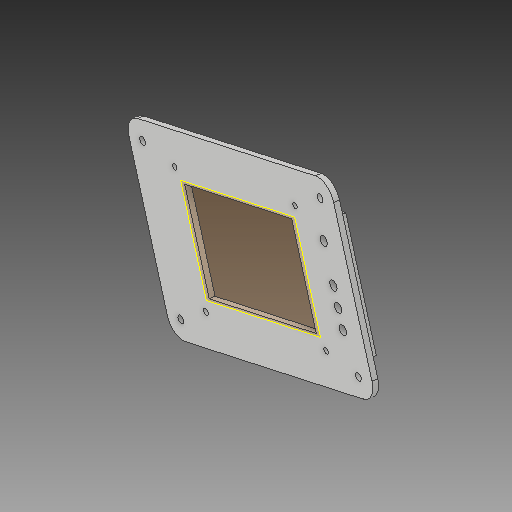
# Autodesk Inventor part: Tampa Painel
Saved by Autodesk Inventor 2019 (Build 230136000, 136)
## iProperties
Created: 2020-05-29
Part Number: Tampa Painel
Material: Generic
Document SubType Name: Modeling
Designer: luiza
Density: 1 g/cm^3
Appearance: Default
Author: luiza
Autodesk Inventor part; units mm, degrees
ref_plane "YZ Plane" through (0, 0, 0) normal (1, 0, 0) x (0, 1, 0)
ref_plane "XZ Plane" through (0, 0, 0) normal (0, 1, 0) x (-1, 0, 0)
ref_plane "XY Plane" through (0, 0, 0) normal (0, 0, 1) x (1, 0, 0)
ref_plane "Work Plane2" through (-1670.9187, -273.4985, -5718.1339) normal (-0.1475237, -0.0099436, 0.9890085) x (0.9373069, 0.3178125, 0.143007)
sketch "Sketch2" plane through (-1670.9187, -273.4985, -5718.1339) normal (-0.1475237, -0.0099436, 0.9890085) x (0.9373069, 0.3178125, 0.143007)
  line L0 (0, 51) -> (78, 51) construction
  line L1 (78, 51) -> (78, 0) construction
  line L2 (78, 0) -> (0, 0) construction
  line L3 (0, 0) -> (0, 51) construction
  line L4 (78.2, 51.2) -> (-0.2, 51.2)
  line L5 (-0.2, 51.2) -> (-0.2, -0.2)
  line L6 (-0.2, -0.2) -> (78.2, -0.2)
  line L7 (78.2, -0.2) -> (78.2, 51.2)
  line L8 (-26, 75.5) -> (104, 75.5)
  line L9 (114, 65.5) -> (114, -14.5)
  line L10 (-26, -24.5) -> (104, -24.5)
  line L11 (-36, 65.5) -> (-36, -14.5)
  line L12 (-7.5, 75.5) -> (-7.5, -24.5) construction
  circle A0 centre (1109.8895, -39.0871) radius 1.5 projected
  circle A1 centre (1103.525, -103.7747) radius 1.5 projected
  circle A2 centre (1191.1021, -112.3913) radius 1.5 projected
  circle A3 centre (1197.4666, -47.7037) radius 1.5 projected
  arc A4 (-26, 75.5) -> (-36, 65.5) centre (-26, 65.5) ccw
  arc A5 (114, 65.5) -> (104, 75.5) centre (104, 65.5) ccw
  arc A6 (104, -24.5) -> (114, -14.5) centre (104, -14.5) ccw
  arc A7 (-36, -14.5) -> (-26, -24.5) centre (-26, -14.5) ccw
  circle A8 centre (99.75, 5.5) radius 2.5
  circle A9 centre (99.75, 15.5) radius 2.5
  circle A10 centre (99.75, 25.5) radius 2.5
  circle A11 centre (99.6463, 45.4997) radius 2.5
  point P0 (2470.8183, -483.0734)
  point P1 (114, 75.5)
  point P2 (114, -24.5)
  point P3 (114, 25.5)
  point P4 (78, 25.5)
  point P5 (-36, 75.5)
  point P6 (-36, -24.5)
  point P7 (39, 75.5)
  point P8 (39, 51)
  dimension "d1" = 0.2
  dimension "d3" = 100
  dimension "d4" = 150
  dimension "d12" = 10
  dimension "d17" = 5
  dimension "d18" = 5
  dimension "d19" = 5
  dimension "d21" = 5
  dimension "d22" = 5
  dimension "d23" = 14.25
  dimension "d24" = 40
  dimension "d27" = 5
  dimension "d29" = 15
  constraints: 26 end point, 10 point on line, 8 centre point, 8 point on circle, 8 tangent, 4 midpoint, 4 parallel, 3 equal radius, 3 horizontal, 3 perpendicular, 2 vertical, 1 horizontal alignment, 1 vertical alignment, 5 other
  measures "d1" distance between parallel lines of L0 L4
  measures "d3" distance between parallel lines of L8 L10
  measures "d4" distance between parallel lines of L11 L9
  measures "d12" radius of A4
  measures "d17" diameter of A10
  measures "d18" diameter of A9
  measures "d19" diameter of A8
  measures "d23" distance from line of L9 A9.centre
  measures "d24" distance from line of L10 A9.centre
  measures "d27" diameter of A11
extrude "Extrusion2" add sketch "Sketch2" against normal blind 3 contours L8 A5 L9 A6 L10 A7 L11 A4
sketch "Sketch3" plane through (-1670.9187, -273.4985, -5718.1339) normal (-0.1475237, -0.0099436, 0.9890085) x (0.9373069, 0.3178125, 0.143007)
  line L0 (-26, -7.5) -> (-33, -7.5) projected
  line L1 (-33, -7.5) -> (-33, 58.5) projected
  line L2 (-33, 58.5) -> (-26, 58.5) projected
  line L3 (-19, 65.5) -> (-19, 72.5) projected
  line L4 (-19, 72.5) -> (97, 72.5) projected
  line L5 (97, 72.5) -> (97, 65.5) projected
  line L6 (104, 58.5) -> (111, 58.5) projected
  line L7 (111, 58.5) -> (111, -7.5) projected
  line L8 (111, -7.5) -> (104, -7.5) projected
  line L9 (97, -14.5) -> (97, -21.5) projected
  line L10 (97, -21.5) -> (-19, -21.5) projected
  line L11 (-19, -21.5) -> (-19, -14.5) projected
  line L12 (-36, -14.5) -> (-36, 65.5) projected
  line L13 (104, -24.5) -> (-26, -24.5) projected
  line L14 (114, 65.5) -> (114, -14.5) projected
  line L15 (-26, 75.5) -> (104, 75.5) projected
  circle A0 centre (-26, 65.5) radius 2 projected
  circle A1 centre (104, -14.5) radius 2 projected
  circle A2 centre (-26, -14.5) radius 2 projected
  circle A3 centre (104, 65.5) radius 2 projected
  arc A4 (-26, 58.5) -> (-19, 65.5) centre (-26, 65.5) ccw projected
  arc A5 (97, 65.5) -> (104, 58.5) centre (104, 65.5) ccw projected
  arc A6 (104, -7.5) -> (97, -14.5) centre (104, -14.5) ccw projected
  arc A7 (-19, -14.5) -> (-26, -7.5) centre (-26, -14.5) ccw projected
  arc A8 (-36, -14.5) -> (-26, -24.5) centre (-26, -14.5) ccw projected
  arc A9 (104, -24.5) -> (114, -14.5) centre (104, -14.5) ccw projected
  arc A10 (114, 65.5) -> (104, 75.5) centre (104, 65.5) ccw projected
  arc A11 (-26, 75.5) -> (-36, 65.5) centre (-26, 65.5) ccw projected
  point P0 (2470.8183, -483.0734)
extrude "Extrusion3" cut sketch "Sketch3" against normal through all contours A0 | A1 | A2 | A3
sketch "Sketch4" plane through (-1670.4761, -273.4687, -5721.1009) normal (0.1475237, 0.0099436, -0.9890085) x (-0.9373069, -0.3178125, -0.143007)
  line L0 (26, -7.5) -> (33, -7.5) projected
  line L1 (33, -7.5) -> (33, 58.5) projected
  line L2 (33, 58.5) -> (26, 58.5) projected
  line L3 (19, 65.5) -> (19, 72.5) projected
  line L4 (19, 72.5) -> (-97, 72.5) projected
  line L5 (-97, 72.5) -> (-97, 65.5) projected
  line L6 (-104, 58.5) -> (-111, 58.5) projected
  line L7 (-111, 58.5) -> (-111, -7.5) projected
  line L8 (-111, -7.5) -> (-104, -7.5) projected
  line L9 (-97, -14.5) -> (-97, -21.5) projected
  line L10 (-97, -21.5) -> (19, -21.5) projected
  line L11 (19, -21.5) -> (19, -14.5) projected
  line L12 (36, -14.5) -> (36, 65.5) projected
  line L13 (-104, -24.5) -> (26, -24.5) projected
  line L14 (-114, 65.5) -> (-114, -14.5) projected
  line L15 (26, 75.5) -> (-104, 75.5) projected
  circle A0 centre (26, 65.5) radius 2 projected
  circle A1 centre (-104, -14.5) radius 2 projected
  circle A2 centre (26, -14.5) radius 2 projected
  circle A3 centre (-104, 65.5) radius 2 projected
  arc A4 (19, 65.5) -> (26, 58.5) centre (26, 65.5) ccw projected
  arc A5 (-104, 58.5) -> (-97, 65.5) centre (-104, 65.5) ccw projected
  arc A6 (-97, -14.5) -> (-104, -7.5) centre (-104, -14.5) ccw projected
  arc A7 (26, -7.5) -> (19, -14.5) centre (26, -14.5) ccw projected
  arc A8 (26, -24.5) -> (36, -14.5) centre (26, -14.5) ccw projected
  arc A9 (-114, -14.5) -> (-104, -24.5) centre (-104, -14.5) ccw projected
  arc A10 (-104, 75.5) -> (-114, 65.5) centre (-104, 65.5) ccw projected
  arc A11 (36, 65.5) -> (26, 75.5) centre (26, 65.5) ccw projected
  line L16 (-96, 65.5) -> (-96, 71.5)
  line L17 (-96, 71.5) -> (18, 71.5)
  line L18 (18, 71.5) -> (18, 65.5)
  arc A12 (18, 65.5) -> (26, 57.5) centre (26, 65.5) ccw
  line L19 (26, 57.5) -> (32, 57.5)
  line L20 (32, 57.5) -> (32, -6.5)
  line L21 (32, -6.5) -> (26, -6.5)
  arc A13 (26, -6.5) -> (18, -14.5) centre (26, -14.5) ccw
  line L22 (18, -14.5) -> (18, -20.5)
  line L23 (18, -20.5) -> (-96, -20.5)
  line L24 (-96, -20.5) -> (-96, -14.5)
  arc A14 (-96, -14.5) -> (-104, -6.5) centre (-104, -14.5) ccw
  line L25 (-104, -6.5) -> (-110, -6.5)
  line L26 (-110, -6.5) -> (-110, 57.5)
  line L27 (-110, 57.5) -> (-104, 57.5)
  arc A15 (-104, 57.5) -> (-96, 65.5) centre (-104, 65.5) ccw
  line L28 (-93, 65.5) -> (-93, 68.5)
  line L29 (-93, 68.5) -> (15, 68.5)
  line L30 (15, 68.5) -> (15, 65.5)
  arc A16 (15, 65.5) -> (26, 54.5) centre (26, 65.5) ccw
  line L31 (26, 54.5) -> (29, 54.5)
  line L32 (29, 54.5) -> (29, -3.5)
  line L33 (29, -3.5) -> (26, -3.5)
  arc A17 (26, -3.5) -> (15, -14.5) centre (26, -14.5) ccw
  line L34 (15, -14.5) -> (15, -17.5)
  line L35 (15, -17.5) -> (-93, -17.5)
  line L36 (-93, -17.5) -> (-93, -14.5)
  arc A18 (-93, -14.5) -> (-104, -3.5) centre (-104, -14.5) ccw
  line L37 (-104, -3.5) -> (-107, -3.5)
  line L38 (-107, -3.5) -> (-107, 54.5)
  line L39 (-107, 54.5) -> (-104, 54.5)
  arc A19 (-104, 54.5) -> (-93, 65.5) centre (-104, 65.5) ccw
  point P0 (-2470.8183, -483.0734)
  point P1 (26, 65.5)
  point P2 (-104, 65.5)
  point P3 (-104, -14.5)
  point P4 (26, -14.5)
  dimension "d38" = 1
  dimension "d39" = 3
  constraints: 48 end point, 16 point on circle, 8 centre point, 30 other
  measures "d38" radial gap between concentric circles of A5 A15
  measures "d39" radial gap between concentric circles of A15 A19
extrude "Extrusion4" add sketch "Sketch4" along normal blind 4 contours L16 L17 L18 A12 L19 L20 L21 A13 L22 L23 L24 A14 L25 L26 L27 A15
sketch "Sketch5" plane through (-1670.9187, -273.4985, -5718.1339) normal (-0.1475237, -0.0099436, 0.9890085) x (0.9373069, 0.3178125, 0.143007)
  circle A0 centre (-5, -7) radius 1.7
  circle A1 centre (83, -7) radius 1.515
  circle A2 centre (83, 58) radius 1.515
  circle A3 centre (-5, 58) radius 1.5
  point P0 (2470.8183, -483.0734)
  constraints: 4 centre point
extrude "Extrusion5" cut sketch "Sketch5" against normal up to surface (3 mm away)
body "Solid2"
